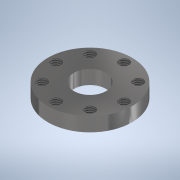
# Autodesk Inventor part: FreeHorn
Saved by Autodesk Inventor 2020.4 (Build 244396000, 396)
## iProperties
Part Number: FreeHorn
Material: アルミニウム 2014-T4
Document SubType Name: Modeling
Designer: Masato Kubotera
Density: 2.8 g/cm^3
Appearance: 半つや出し
Mass: 2.533 g
Surface Area: 10.4083 cm^2
Volume: 0.938147 cm^3
Description: ReadyMade
Catalog Web Link: https://kondo-robot.com/product/02137
Author: Masato Kubotera
Autodesk Inventor part; units mm, degrees
ref_plane "YZ Plane" through (0, 0, 0) normal (1, 0, 0) x (0, 1, 0)
ref_plane "XZ Plane" through (0, 0, 0) normal (0, 1, 0) x (-1, 0, 0)
ref_plane "XY Plane" through (0, 0, 0) normal (0, 0, 1) x (1, 0, 0)
sketch "スケッチ1" plane through (0, 0, 0) normal (0, 0, 1) x (1, 0, 0)
  circle A0 centre (0, 0) radius 10.5
  circle A1 centre (0, 0) radius 4
  line L0 (0, 8.5) -> (0, 0) construction
  point P0 (-6.0104, 6.0104)
  point P1 (-8.5, 0)
  point P2 (-6.0104, -6.0104)
  point P3 (0, -8.5)
  point P4 (6.0104, -6.0104)
  point P5 (8.5, 0)
  point P6 (6.0104, 6.0104)
  dimension "d0" = 21
  dimension "d1" = 8
  dimension "d16" = 8.5
  dimension "d19" = 360
  constraints: 3 coincident, 2 centre point, 2 end point, 1 vertical, 9 other
  measures "d0" diameter of A0
  measures "d1" diameter of A1
  measures "d16" distance of L0.start L0.end
extrude "押し出し1" add sketch "スケッチ1" along normal blind 3.5
hole "穴2" at (0, 8.5, 0) at (-6.0104, 6.0104, 0) at (-8.5, 0, 0) at (-6.0104, -6.0104, 0) at (0, -8.5, 0) at (6.0104, -6.0104, 0) at (8.5, 0, 0) at (6.0104, 6.0104, 0) direction (0, 0, 1) diameter 2.459 end through all countersink diameter 4 countersink angle 90 thread size "M3x0.5" class "6H" standard "ISO Metric profile"
